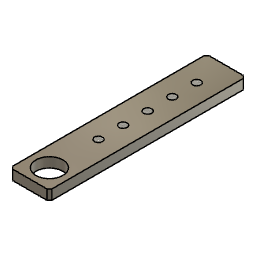
lift spring mount v1 (Autodesk Fusion 360 design; units mm, degrees)
Autodesk Fusion 360 part; units mm, degrees
note: some values were not read from the file. Set by a fixed rule: the direction of a hole.
sketch "Sketch1" plane through (0, 0, 0) normal (0, 1, 0) x (1, 0, 0)
  line L0 (-4, 40) -> (4, 40)
  line L1 (4, 40) -> (4, 0)
  line L2 (4, 0) -> (-4, 0)
  line L3 (-4, 0) -> (-4, 40)
  point P0 (0, 4)
  point P1 (0, 14)
  dimension "d1" = 8
  dimension "d2" = 40
  dimension "d3" = 4
  dimension "d4" = 10
  constraint horizontal L0
  constraint vertical L1
  constraint horizontal L2
  constraint vertical L3
  constraint midpoint origin L2
  constraint vertical origin P0
  constraint vertical P0 P1
  measures "d1" distance of L0.start L0.end
  measures "d2" distance of L0.start L2.end
  measures "d3" distance of L2 P0
  measures "d4" distance of P0 P1
extrude "Extrude1" add sketch "Sketch1" along normal blind 2
hole "Hole1" at (0, 0, -4) direction (0, 1, 0) diameter 5.5 depth 16 tip angle 118
hole "Hole2" at (0, 0, -14) direction (0, 1, 0) diameter 1.623 depth 16 tip angle 118
thread "Thread1" "ISO Metric profile 2.0 M2x0.4 6H" thread offset 0 thread depth 10
pattern_linear "R-Pattern1" count 5 spacing 5 along (0, 0, -1) of "Hole2"
chamfer "Chamfer1" distance 0.5 angle 45 4 edges at (4, 1, 0) (-4, 1, 0) (4, 1, -40) (-4, 1, -40)
